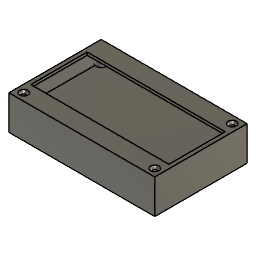
2004A_display_case (Autodesk Fusion 360 design; units mm, degrees)
Autodesk Fusion 360 part; units mm, degrees
note: some values were not read from the file. Set by a fixed rule: which sketch regions a step uses.
sketch "Sketch1" plane through (0, 0, 0) normal (0, 0, 1) x (1, 0, 0)
  line L0 (0, 0) -> (98, 0)
  line L1 (98, 0) -> (98, 60)
  line L2 (98, 60) -> (0, 60)
  line L3 (0, 60) -> (0, 0)
  line L4 (-0.8, -0.8) -> (98.8, -0.8)
  line L5 (98.8, -0.8) -> (98.8, 60.8)
  line L6 (98.8, 60.8) -> (-0.8, 60.8)
  line L7 (-0.8, 60.8) -> (-0.8, -0.8)
  line L8 (-2.8, -2.8) -> (100.8, -2.8)
  line L9 (100.8, -2.8) -> (100.8, 62.8)
  line L10 (100.8, 62.8) -> (-2.8, 62.8)
  line L11 (-2.8, 62.8) -> (-2.8, -2.8)
  circle A0 centre (95.5, 57.5) radius 1.3
  circle A1 centre (95.5, 2.5) radius 1.3
  circle A2 centre (2.5, 2.5) radius 1.3
  circle A3 centre (2.5, 2.5) radius 3.5
  circle A4 centre (95.5, 57.5) radius 3.5
  circle A5 centre (95.5, 2.5) radius 3.5
  line L12 (0, 10) -> (98, 10)
  line L13 (98, 10) -> (98, 50)
  line L14 (98, 50) -> (0, 50)
  line L15 (0, 50) -> (0, 10)
  circle A6 centre (2.5, 57.5) radius 3.5
  point P0 (10, 57.5)
  dimension "d7" = 98
  dimension "d8" = 60
  dimension "d9" = 0.8
  dimension "d10" = 2
  dimension "d11" = 2.6
  dimension "d12" = 2.6
  dimension "d14" = 2.6
  dimension "d17" = 2.5
  dimension "d18" = 2.5
  dimension "d19" = 2.5
  dimension "d20" = 2.5
  dimension "d23" = 7
  dimension "d24" = 7
  dimension "d25" = 7
  dimension "d58" = 2.5
  dimension "d59" = 2.5
  dimension "d60" = 10
  dimension "d61" = 10
  dimension "d62" = 10
  dimension "d65" = 2.5
  dimension "d66" = 7
  dimension "d67" = 2.5
  dimension "d68" = 2.5
  constraint coincident L0.start L3.end
  constraint horizontal L0
  constraint vertical L1
  constraint horizontal L2
  constraint vertical L3
  constraint concentric A2 A3
  constraint concentric A0 A4
  constraint concentric A1 A5
  constraint horizontal L12
  constraint vertical L13
  constraint horizontal L14
  constraint vertical L15
  constraint coincident L1 L13.end
  constraint coincident L3 L12.start
  measures "d7" distance of L1 L3
  measures "d8" distance of L0 L2
  measures "d11" diameter of A0
  measures "d12" diameter of A1
  measures "d14" diameter of A2
  measures "d17" distance of L2 A0.centre
  measures "d18" distance of L1 A0.centre
  measures "d19" distance of L1 A1.centre
  measures "d20" distance of L0 A1.centre
  measures "d23" diameter of A3
  measures "d24" diameter of A4
  measures "d25" diameter of A5
  measures "d58" distance of P0 L2
  measures "d59" distance of L0 A2.centre
  measures "d60" distance of P0 L3
  measures "d61" distance of L2 L14
  measures "d62" distance of L0 L12
  measures "d65" distance of L3 A2.centre
  measures "d66" diameter of A6
  measures "d67" distance of L2 A6.centre
  measures "d68" distance of L3 A6.centre
extrude "Extrude4" add sketch "Sketch1" along normal blind 9.6 contours L0 L3 A3 | L0 L3 L4 L7 A3 | L0 L3 A3 | L0 L4 A3 | L3 L7 A3 | L0 L1 L3 A3 A5 L12 | L0 L4 A3 A5 | L4 A3 | L3 L7 A3 L15 A6 | L7 A3 | L0 L1 A5 | L0 L4 A5 | L0 L1 A5 | L0 L1 L4 L5 A5 | L1 L5 A5 | L1 L5 A4 A5 L13 | L4 A5 | L1 L2 L3 A4 L14 A6 | L7 A6 | L3 L7 A6 | L5 A5 | L2 L3 A6 | L2 L3 L6 L7 A6 | L1 L5 A4 | L5 A4 | L2 L3 A6 | L1 L2 A4 | L1 L2 L5 L6 A4 | L2 L6 A6 | L2 L6 A4 A6 | L1 L2 A4 | L2 L6 A4 | L6 A6 | L6 A4 | L8 L9 L10 L11 makes body 1
extrude "Extrude6" cut sketch "Sketch1" along normal blind 7.6 contours L0 L3 L4 L7 A3 | L0 L1 L3 A3 A5 L12 | L0 L4 A3 A5 | L3 L7 A3 L15 A6 | L1 L3 L12 L13 L14 L15 | L0 L1 A5 | L0 L1 L4 L5 A5 | L1 L5 A4 A5 L13 | L1 L2 L3 A4 L14 A6 | L2 L3 L6 L7 A6 | L2 L3 A6 | L1 L2 L5 L6 A4 | L2 L6 A4 A6 | L1 L2 A4 picked at (97.9832, 0.0168) picked at (0.0168, 59.9832) picked at (97.9832, 59.9832) bodies 1
extrude "Extrude7" add sketch "Sketch1" against normal blind 14.8 contours L4 A3 | L7 A3 | L4 A5 | L7 A6 | L5 A5 | L5 A4 | L6 A6 | L6 A4 | L8 L9 L10 L11 bodies 1
extrude "Extrude8" add sketch "Sketch1" against normal blind 3.3 separate body contours L0 L3 A3 | L0 L3 A3 | L0 L1 L3 A3 A5 L12 | L0 L1 A5 | L1 L3 L12 L13 L14 L15 | L0 L1 A5 | L1 L2 L3 A4 L14 A6 | L2 L3 A6 | L2 L3 A6 | L1 L2 A4 | L1 L2 A4 makes body 2
extrude "Extrude9" cut sketch "Sketch1" against normal blind 1.3 contours L0 L3 A3 | L0 L1 L3 A3 A5 L12 | L1 L3 L12 L13 L14 L15 | L0 L1 A5 | L1 L2 L3 A4 L14 A6 | L2 L3 A6 | L2 L3 A6 | L1 L2 A4 picked at (0.0168, 0.0168) picked at (97.9832, 0.0168) picked at (97.9832, 59.9832) bodies 2
sketch "Sketch2" plane through (-2.8, 0, 0) normal (-1, 0, 0) x (0, -1, 0)
  line L0 (2.8, -14.8) -> (2.8, 9.6)
  line L1 (2.8, 9.6) -> (-62.8, 9.6)
  line L2 (-62.8, 9.6) -> (-62.8, -14.8)
  line L3 (-62.8, -14.8) -> (2.8, -14.8)
  line L4 (-48.5, -5) -> (-35.5, -5)
  line L5 (-35.5, -5) -> (-35.5, -13)
  line L6 (-35.5, -13) -> (-48.5, -13)
  line L7 (-48.5, -13) -> (-48.5, -5)
  line L8 (-6, 0) -> (0.8, 0)
  point P0 (-57.5, 0)
  dimension "d49" = 8
  dimension "d50" = 13
  dimension "d63" = 9
  dimension "d64" = 5
  constraint horizontal L4
  constraint vertical L5
  constraint horizontal L6
  constraint vertical L7
  measures "d49" distance of L4 L6
  measures "d50" distance of L5 L7
  measures "d63" distance of L7 P0
  measures "d64" distance of L4 origin
extrude "Extrude10" cut sketch "Sketch2" against normal blind 2 contours L4 L5 L6 L7 bodies 1
chamfer "Chamfer1" distance 1.6 angle 45 3 edges at (94.288, 57.9701, 9.6) (94.288, 2.9701, 9.6) (1.288, 2.9701, 9.6) on bodies 1
